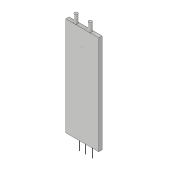
# Autodesk Inventor part: ir sensor
Saved by Autodesk Inventor 2019 (Build 230136000, 136)
## iProperties
Created: 2019-10-10
Part Number: ir sensor
Material: Generic
Document SubType Name: Modeling
Designer: Admin
Density: 1 g/cm^3
Appearance: Default
Author: Admin
Autodesk Inventor part; units mm, degrees
ref_plane "YZ Plane" through (0, 0, 0) normal (1, 0, 0) x (0, 1, 0)
ref_plane "XZ Plane" through (0, 0, 0) normal (0, 1, 0) x (-1, 0, 0)
ref_plane "XY Plane" through (0, 0, 0) normal (0, 0, 1) x (1, 0, 0)
sketch "Sketch1" plane through (0, 0, 0) normal (0, 0, 1) x (1, 0, 0)
  line L0 (0, 0.2366) -> (10, 0.2366)
  line L1 (10, 0.2366) -> (10, 30.2366)
  line L2 (10, 30.2366) -> (0, 30.2366)
  line L3 (0, 30.2366) -> (0, 0.2366)
  point P0 (0, 0)
  dimension "d0" = 10
  dimension "d1" = 30
  constraints: 8 end point, 2 parallel, 1 horizontal, 1 perpendicular
  measures "d0" distance of L2.end L1.end
  measures "d1" distance of L1.end L0.end
extrude "Extrusion1" add sketch "Sketch1" along normal blind 1
sketch "Sketch2" plane through (0, 30.2366, 0) normal (0, 1, 0) x (1, 0, 0)
  line L0 (0, 0) -> (0, -1) projected
  line L1 (0, -0.5) -> (10, -0.5)
  line L2 (0, 0) -> (10, 0) projected
  line L3 (2.646, -1) -> (2.646, 0.5163)
  line L4 (6.9484, -1) -> (6.9484, 0)
  circle A0 centre (2.646, -0.5) radius 0.5
  circle A1 centre (6.9484, -0.5) radius 0.5
  dimension "d4" = 1
  constraints: 6 end point, 3 point on line, 2 centre point, 2 midpoint, 2 perpendicular, 1 parallel, 1 tangent
  measures "d4" diameter of A1
extrude "Extrusion2" add sketch "Sketch2" along normal blind 2.5 contours A0 L1 L3 | L3 L1 A0 | L1 L3 A0 | A1 L1 L4 | L4 L1 A1 | L1 A0 L3 | L4 A1 L1 | L1 A1 L4
sketch "Sketch3" plane through (0, 0, 0) normal (0, 0, -1) x (-1, 0, 0)
  line L0 (-3.175, 1.5875) -> (-3.175, -3.4125)
  line L1 (-5, 1.5875) -> (-5, -3.4125)
  line L2 (-7.0347, 1.5875) -> (-7.0347, -3.4125)
  point P0 (0, 0)
  dimension "d7" = 5
  dimension "d8" = 5
  dimension "d9" = 5
  constraints: 6 end point, 3 vertical
  measures "d7" distance of L0.start L0.end
  measures "d8" distance of L1.start L1.end
  measures "d9" distance of L2.start L2.end
sketch "Sketch4" plane through (0, 0, 1) normal (0, 0, 1) x (1, 0, 0)
  line L0 (4.7625, 30.1625) -> (4.7625, 25.1625)
  circle A0 centre (4.7625, 25.1625) radius 0.05
  point P0 (0, 0)
  dimension "d10" = 5
  dimension "d11" = 0.1
  constraints: 2 end point, 1 centre point, 1 coincident, 1 vertical
  measures "d10" distance of L0.start L0.end
  measures "d11" diameter of A0
extrude "Extrusion3" cut sketch "Sketch4" against normal through all
body "Solid1"
